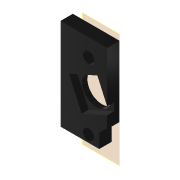
# Autodesk Inventor part: 30_Linear_Stage_NEMA11_baseholder_bayonetmount_objective_autofocus_kes400_camerabracket_underAnAngle
Saved by Autodesk Inventor 2022 (Build 260153000, 153)
## iProperties
Created: 2023-05-15
Part Number: 30_Linear_Stage_NEMA11_baseholder_bayonetmount_objective_autofocus_kes400_camerabracket_underAnAngle
Material: Generisch
Document SubType Name: Modeling
Designer: diederichbenedict
Density: 1 g/cm^3
Appearance: Glatt - Schwarz
Author: diederichbenedict
Autodesk Inventor part; units mm, degrees
ref_plane "YZ Plane" through (0, 0, 0) normal (1, 0, 0) x (0, 1, 0)
ref_plane "XZ Plane" through (0, 0, 0) normal (0, 1, 0) x (-1, 0, 0)
ref_plane "Arbeitsebene1" through (0, 0, 0) normal (0, 0, 1) x (1, 0, 0)
sketch "Skizze1" plane through (0, 0, 0) normal (0, 0, 1) x (1, 0, 0)
  line L0 (-7.7466, -5.9177) -> (-1.7466, -5.9177)
  line L1 (-1.7466, -5.9177) -> (-1.7466, 2.0823)
  line L2 (-1.7466, 2.0823) -> (-7.7466, 2.0823)
  line L3 (-7.7466, 2.0823) -> (-7.7466, -5.9177)
  line L4 (-7.7466, -5.9177) -> (-1.7466, 2.0823) construction
  line L5 (-1.7466, -5.9177) -> (-7.7466, 2.0823) construction
  line L6 (-7.7466, -5.9177) -> (-1.7466, -5.9177)
  line L7 (-1.7466, -5.9177) -> (-1.7466, -3.9177)
  line L8 (-1.7466, -3.9177) -> (-7.7466, -3.9177)
  line L9 (-7.7466, -3.9177) -> (-7.7466, -5.9177)
  circle A0 centre (-4.7466, -1.9177) radius 1.6
  line L10 (0.5034, 22.0823) -> (-10.1632, 22.0823)
  line L11 (-10.1632, 22.0823) -> (-10.1632, 2.0823)
  line L12 (-10.1632, 2.0823) -> (0.5034, 2.0823)
  line L13 (0.5034, 2.0823) -> (0.5034, 22.0823)
  line L14 (0.5034, 22.0823) -> (-10.1632, 2.0823) construction
  line L15 (-10.1632, 22.0823) -> (0.5034, 2.0823) construction
  circle A1 centre (-4.7466, 17.0823) radius 1.6
  circle A2 centre (-4.4966, 8.0823) radius 4.1
  line L16 (-7.7466, -5.9177) -> (-10.1632, -5.9177)
  line L17 (-10.1632, -5.9177) -> (-10.1632, 2.0823)
  line L18 (-10.1632, 2.0823) -> (-7.7466, 2.0823)
  line L19 (-7.7466, 2.0823) -> (-7.7466, -5.9177)
  line L20 (-10.1632, -5.9177) -> (-12.7262, -5.9177)
  line L21 (-12.7262, -5.9177) -> (-12.7262, 22.0823)
  line L22 (-12.7262, 22.0823) -> (-10.1632, 22.0823)
  line L23 (-10.1632, 22.0823) -> (-10.1632, -5.9177)
  point P0 (0, 0)
  point P1 (-7.7466, -3.9177)
  point P2 (-4.8299, 12.0823)
  point P3 (-1.7466, 2.0823)
  point P4 (-7.7466, 2.0823)
  point P5 (-4.7466, 2.0823)
  dimension "d0" = 6
  dimension "d1" = 8
  dimension "d10" = 2
  dimension "d11" = 3.2
  dimension "d12" = 20
  dimension "d13" = 3.2
  dimension "d14" = 19
  dimension "d15" = 8.2
  dimension "d44" = 0
  dimension "d45" = 5.25
  dimension "d46" = 9
  dimension "d53" = 0.25
  constraints: 49 end point, 10 parallel, 5 horizontal, 5 perpendicular, 4 midpoint, 3 centre point, 2 point on line
  measures "d0" distance of L2.end L1.end
  measures "d1" distance of L1.end L0.end
  measures "d10" distance of L7.end L6.end
  measures "d11" diameter of A0
  measures "d12" distance between parallel lines of L12 L10
  measures "d13" diameter of A1
  measures "d14" distance of A0.centre A1.centre
  measures "d15" diameter of A2
  measures "d44" horizontal distance of A0.centre A1.centre
  measures "d45" distance from line of L13 A1.centre
  measures "d46" vertical distance of A2.centre A1.centre
  measures "d53" horizontal distance of A2.centre A1.centre
ref_plane "Arbeitsebene2" through (-9.2536, 3.4368, 4) normal (0, 0, 1) x (1, -0.0003, 0)
extrude "Extrusion1" add sketch "Skizze1" along normal blind 1.5 contours L16 L17 L12 L3 | L3 L2 L1 L8 | L20 L21 L22 L11 L17 | L12 L11 L10 L13 L2
sketch "Skizze4" plane through (0, 0, 1.5) normal (0, 0, 1) x (1, 0, 0)
  line L0 (-55.6662, 35.6355) -> (-7.4062, 35.6355) construction
  line L1 (-7.4062, 35.6355) -> (-7.4062, -28.7112) construction
  line L2 (-7.4062, -28.7112) -> (-55.6662, -28.7112) construction
  line L3 (-55.6662, -28.7112) -> (-55.6662, 35.6355) construction
  line L4 (-34.8105, 18.9517) -> (-34.8105, 11.3513)
  line L5 (-34.8105, 11.3513) -> (-29.4903, 14.6086)
  line L6 (-1.7466, -3.9177) -> (-1.7466, 2.0823) projected
  line L7 (-1.7466, 2.0823) -> (0.5034, 2.0823) projected
  line L8 (0.5034, 2.0823) -> (0.5034, 22.0823) projected
  line L9 (-7.7466, -5.9177) -> (-7.7466, -3.9177) projected
  line L10 (-7.7466, -3.9177) -> (-1.7466, -3.9177) projected
  circle A0 centre (-4.7466, 17.0823) radius 1.6 projected
  circle A1 centre (-4.4966, 8.0823) radius 4.1 projected
  circle A2 centre (-4.7466, -1.9177) radius 1.6 projected
  line L11 (1.3127, 5.8523) -> (-2.2666, 13.8915)
  line L12 (-2.2666, 13.8915) -> (-10.3058, 10.3122)
  line L13 (-10.3058, 10.3122) -> (-6.7265, 2.273)
  line L14 (-6.7265, 2.273) -> (1.3127, 5.8523)
  line L15 (1.3127, 5.8523) -> (-10.3058, 10.3122) construction
  line L16 (-2.2666, 13.8915) -> (-6.7265, 2.273) construction
  line L17 (1.3127, 5.8523) -> (10.1127, 5.8523) construction
  line L18 (0.5034, 22.0823) -> (-12.7262, 22.0823) projected
  line L19 (-12.7262, 22.0823) -> (-12.7262, -5.9177) projected
  line L20 (-12.7262, -5.9177) -> (-7.7466, -5.9177) projected
  line L21 (-7.7466, -3.9177) -> (-1.7466, -3.9177) projected
  line L22 (-7.7466, -3.9177) -> (-12.7262, -3.9177)
  line L23 (-12.7262, 22.0823) -> (-12.7262, -5.9177) projected
  point P0 (0, 0)
  point P1 (0.5034, 5.492)
  point P2 (0.5034, 7.6699)
  dimension "d40" = 8.8
  dimension "d41" = 114
  dimension "d42" = 8.8
  constraints: 20 end point, 2 midpoint, 2 parallel, 2 perpendicular, 1 equal length, 1 horizontal, 1 point on line, 1 vertical, 2 other
  measures "d40" distance of L11.start L11.end
  measures "d41" angle of L17 L11
  measures "d42" distance of L12.end L11.end
extrude "Extrusion4" add sketch "Skizze4" along normal blind 2 contours L10 L22 L19 L18 L8 L11 L12 L13 L14 L7 L6
chamfer "Fase2" distance 2 angle 45 1 edges at (-1.7466, 2.0823, 1.75)
